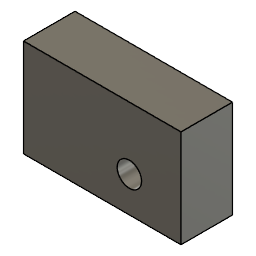
replay (Autodesk Fusion 360 design; units mm, degrees)
Autodesk Fusion 360 part; units mm, degrees
sketch "草图1" plane through (0, 0, 0) normal (0, 0, 1) x (1, 0, 0)
  line L0 (48, 6) -> (48, 42)
  line L1 (48, 42) -> (-10, 42)
  line L2 (-10, 42) -> (-10, 6)
  line L3 (-10, 6) -> (48, 6)
extrude "拉伸1" add sketch "草图1" along normal blind 19
sketch "草图2" plane through (0, 0, 19) normal (0, 0, 1) x (1, 0, 0)
  line L0 (-10, 6) -> (48, 6)
  line L1 (48, 6) -> (48, 42)
  line L2 (48, 42) -> (-10, 42)
  line L3 (-10, 42) -> (-10, 6)
  circle A0 centre (29, 19) radius 4.5
extrude "拉伸2" cut sketch "草图2" against normal through all contours A0
